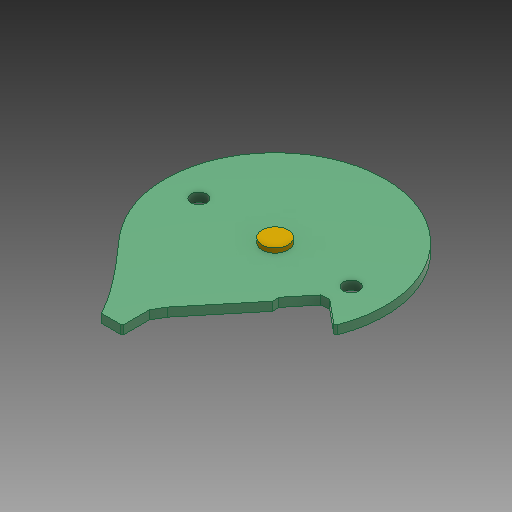
# Autodesk Inventor part: pcb
Saved by Autodesk Inventor 2019 (Build 230136000, 136)
## iProperties
Created: 2016-09-25
Part Number: pcb
Material: Generisch
Document SubType Name: Modeling
Designer: WhoTheHeck
Density: 1 g/cm^3
Appearance: Glatt - dunkelseegrün
Author: WhoTheHeck
Autodesk Inventor part; units mm, degrees
ref_plane "YZ Plane" through (0, 0, 0) normal (1, 0, 0) x (0, 1, 0)
ref_plane "XZ Plane" through (0, 0, 0) normal (0, 1, 0) x (-1, 0, 0)
ref_plane "XY Plane" through (0, 0, 0) normal (0, 0, 1) x (1, 0, 0)
sketch "Skizze1" plane through (0, 0, 0) normal (0, 0, 1) x (1, 0, 0)
  circle A0 centre (0, 0) radius 12.625
  line L0 (31.2972, 39.0088) -> (31.2972, -40.1485) construction
  line L1 (31.2972, -40.1485) -> (-28.0708, -40.1485) construction
  line L2 (-28.0708, -40.1485) -> (-28.0708, 39.0088) construction
  line L3 (-28.0708, 39.0088) -> (31.2972, 39.0088) construction
  line L4 (-10.1529, -7.5039) -> (-9.5297, -8.4617) construction
  line L5 (-9.5297, -8.4617) -> (-6.7964, -11.288) construction
  line L6 (-6.7964, -11.288) -> (-4.1897, -14.7808) construction
  line L7 (-4.1897, -14.7808) -> (-3.5273, -15.9852) construction
  line L8 (-3.5273, -15.9852) -> (-2.9089, -17.0055) construction
  spline S0 degree 4 poles (-10.1529, -7.5039) (-10.1523, -7.5049) (-9.5297, -8.4617) (-6.7964, -11.288) (-4.1897, -14.7808) (-3.5273, -15.9852) (-2.9089, -17.0055) knots 1 1 1 1 1 2 3 4 4 4 4 4
  line L9 (-2.9089, -17.0055) -> (-0.7662, -17.0055)
  arc A1 (-0.7662, -17.0055) -> (-0.5189, -16.9237) centre (-0.7662, -16.5904) ccw
  line L10 (-0.5189, -16.9237) -> (-0.5189, -13.9001)
  line L11 (-0.5189, -13.9001) -> (0.2333, -12.6228)
  line L12 (0.2333, -12.6228) -> (8.5203, -2.5497)
  line L13 (8.809, -2.5289) -> (11.6496, -4.8659)
  line L14 (5.7065, -5.97) -> (5.6548, -5.2536)
  line L15 (5.6548, -5.2536) -> (7.8388, -2.5989)
  line L16 (7.8388, -2.5989) -> (8.809, -2.5289)
  dimension "d0" = 25.25
  constraints: 16 end point, 6 point on circle, 2 centre point, 2 coincident, 2 perpendicular, 2 point on line, 1 horizontal, 1 tangent, 1 vertical, 6 other
  measures "d0" diameter of A0
extrude "Extrusion1" add sketch "Skizze1" along normal blind 1 contours A0 L13 L16 L15 L14 L12 | A0 L11 L10 A1 L9 S0
fillet "Rundung1" radius 0.2 2 edges at (11.6496, -4.8659, 0.5) (8.5203, -2.5497, 0.5)
sketch "Skizze2" plane through (0, 0, 1) normal (0, 0, 1) x (1, 0, 0)
  circle A0 centre (0, 0) radius 1.5
  dimension "d46" = 3
  constraints: 1 centre point, 1 coincident
  measures "d46" diameter of A0
extrude "Extrusion2" add sketch "Skizze2" along normal blind 0.5
sketch "Skizze3" plane through (0, 0, 1) normal (0, 0, 1) x (1, 0, 0)
  line L0 (-8.75, 0) -> (8.75, 0) construction
  circle A0 centre (-8.75, 0) radius 0.9
  circle A1 centre (8.75, 0) radius 0.9
  point P0 (0, 0)
  dimension "d49" = 17.5
  dimension "d50" = 8.75
  dimension "d51" = 1.8
  dimension "d52" = 1.8
  constraints: 2 centre point, 2 coincident, 2 end point, 1 horizontal, 1 midpoint
  measures "d49" distance of L0.start L0.end
  measures "d50" distance of L0.start point (0, 0)
  measures "d51" diameter of A0
  measures "d52" diameter of A1
extrude "Extrusion3" cut sketch "Skizze3" against normal through all
equation "\"d50\" = 0.5 * d49"
equation "\"d52\" = d51"
